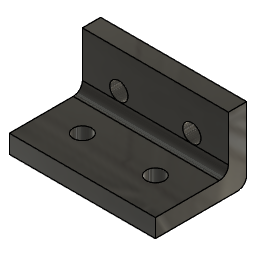
Fully Assembled English Wheel (Autodesk Fusion 360 archive; units mm, degrees)
design "Clamp/Mount Bracket"
Autodesk Fusion 360 part; units mm, degrees
sketch "Sketch1" plane through (0, 0, 0) normal (0, 1, 0) x (1, 0, 0)
  line L0 (50.8, 25.4) -> (-50.8, 25.4)
  line L1 (-50.8, 25.4) -> (-50.8, -25.4)
  line L2 (-50.8, -25.4) -> (50.8, -25.4)
  line L3 (50.8, -25.4) -> (50.8, 25.4)
  line L4 (0, 0) -> (25.4, 0) construction
  line L5 (0, 0) -> (-25.4, 0) construction
  circle A0 centre (-25.4, 0) radius 6.35
  circle A1 centre (25.4, 0) radius 6.35
  dimension "d3" = 101.6
  dimension "d4" = 50.8
  dimension "d5" = 25.4
  dimension "d7" = 12.7
  dimension "d8" = 12.7
  constraint horizontal L0
  constraint perpendicular L0 L1
  constraint parallel L0 L2
  constraint parallel L1 L3
  constraint coincident L4.start L5.start
  constraint horizontal L4
  constraint parallel L4 L5
  constraint coincident L5.end A0.centre
  constraint coincident L4.end A1.centre
  measures "d3" distance of L1.end L2.end
  measures "d4" distance of L0.end L1.end
  measures "d5" distance of L4.start L4.end
  measures "d7" diameter of A0
  measures "d8" diameter of A1
extrude "Extrude1" add sketch "Sketch1" along normal blind 12.7 makes body 1
sketch "Sketch2" plane through (0, 0, 0) normal (0, -1, 0) x (1, 0, 0)
  circle A0 centre (-25.4, 0) radius 6.35
  circle A1 centre (25.4, 0) radius 6.35
  line L0 (50.8, -25.4) -> (50.8, 25.4)
  line L1 (50.8, 25.4) -> (-50.8, 25.4)
  line L2 (-50.8, 25.4) -> (-50.8, -25.4)
  line L3 (-50.8, -25.4) -> (50.8, -25.4)
  line L4 (-50.8, -25.4) -> (50.8, -25.4)
  line L5 (50.8, -25.4) -> (50.8, -12.7)
  line L6 (50.8, -12.7) -> (-50.8, -12.7)
  line L7 (-50.8, -12.7) -> (-50.8, -25.4)
  dimension "d11" = 101.6
  dimension "d12" = 12.7
  constraint horizontal L4
  constraint vertical L5
  constraint horizontal L6
  constraint vertical L7
  constraint coincident L2.end L3.start
  measures "d11" distance of L2.end L0.start
  measures "d12" distance of L0.start L5.end
extrude "Extrude2" add sketch "Sketch2" along normal blind 50.8 contours L0 L2 L3 L4 L5 L6 L7 bodies 1
sketch "Sketch3" plane through (0, 0, -12.7) normal (0, 0, 1) x (-1, 0, 0)
  line L0 (-50.8, 0) -> (50.8, 0)
  line L1 (50.8, 0) -> (50.8, 50.8)
  line L2 (50.8, 50.8) -> (-50.8, 50.8)
  line L3 (-50.8, 50.8) -> (-50.8, 0)
  line L4 (0, 0) -> (0, 50.8) construction
  line L5 (0, 25.4) -> (-25.4, 25.4) construction
  line L6 (0, 25.4) -> (25.4, 25.4) construction
  circle A0 centre (25.4, 25.4) radius 6.35
  circle A1 centre (-25.4, 25.4) radius 6.35
  dimension "d15" = 25.4
  dimension "d16" = 25.4
  dimension "d17" = 12.7
  dimension "d18" = 12.7
  constraint coincident L4.start origin
  constraint midpoint L2 L4.end
  constraint midpoint L4 L5.start
  constraint perpendicular L4 L5
  constraint perpendicular L4 L6
  constraint coincident L6.end A0.centre
  constraint coincident L5.end A1.centre
  measures "d15" distance of L5.start L5.end
  measures "d16" distance of L5.start L6.end
  measures "d17" diameter of A0
  measures "d18" diameter of A1
extrude "Extrude3" cut sketch "Sketch3" against normal blind 43.18 contours A0 | A1 bodies 1
fillet "Fillet1" radius 6.35 2 edges at (0, 0, -12.7) (0, 12.7, -25.4) on bodies 1
copy_body "Body->Comp1" bodies 1 removing the originals makes body 2 in component "Clamp/Mount Bracket"
component "Clamp/Mount Bracket" placed x (1, 0, 0) y (0, 1, 0) z (0, 0, 1) at (0, 0, 0)
equation "d7 = ( 1 / 2 ) * 1 in"
equation "d8 = ( 1 / 2 ) * 1 in"
equation "d9 = ( 1 / 2 ) * 1 in"
equation "d17 = ( 1 / 2 ) * 1 in"
equation "d18 = ( 1 / 2 ) * 1 in"
equation "d22 = ( 1 / 4 ) * 1 in"

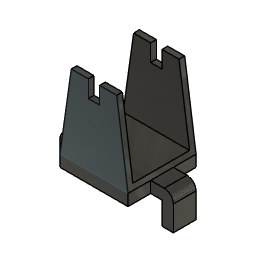
design "Lower Anvil Holder"
Autodesk Fusion 360 part; units mm, degrees
sketch "Sketch1" plane through (0, 0, 0) normal (0, 1, 0) x (1, 0, 0)
  line L0 (19.05, 22.225) -> (-19.05, 22.225)
  line L1 (-19.05, 22.225) -> (-19.05, -22.225)
  line L2 (-19.05, -22.225) -> (19.05, -22.225)
  line L3 (19.05, -22.225) -> (19.05, 22.225)
  line L4 (0, -22.225) -> (12.7, -22.225)
  line L5 (0, -22.225) -> (-12.7, -22.225)
  line L6 (-19.05, 22.225) -> (-12.7, -22.225)
  line L7 (12.7, -22.225) -> (19.05, 22.225)
  line L8 (0, -22.225) -> (3.175, -22.225)
  line L9 (0, -22.225) -> (-3.175, -22.225)
  line L10 (-3.175, -22.225) -> (-3.175, -12.7)
  line L11 (3.175, -22.225) -> (3.175, -12.7)
  line L12 (-3.175, -12.7) -> (3.175, -12.7)
  dimension "d1" = 38.1
  dimension "d2" = 44.45
  constraint horizontal L0
  constraint perpendicular L0 L1
  constraint parallel L0 L2
  constraint parallel L1 L3
  constraint midpoint L2 L4.start
  constraint parallel L2 L4
  constraint coincident L2 L5.end
  constraint coincident L4 L8.end
  constraint coincident L5 L9.end
  constraint perpendicular L5 L10
  constraint perpendicular L2 L11
  measures "d1" distance of L1.end L2.end
  measures "d2" distance of L0.end L1.end
extrude "Extrude1" add sketch "Sketch1" along normal blind 38.1 contours L0 L2 L4 L5 L6 L7 L10 L11 L12 makes body 1
sketch "Sketch2" plane through (0, 0, 0) normal (0, -1, 0) x (1, 0, 0)
  line L0 (-3.175, 12.7) -> (-3.175, 22.225)
  line L1 (-3.175, 22.225) -> (-12.7, 22.225)
  line L2 (-12.7, 22.225) -> (-19.05, -22.225)
  line L3 (-19.05, -22.225) -> (19.05, -22.225)
  line L4 (19.05, -22.225) -> (12.7, 22.225)
  line L5 (12.7, 22.225) -> (3.175, 22.225)
  line L6 (3.175, 22.225) -> (3.175, 12.7)
  line L7 (3.175, 12.7) -> (-3.175, 12.7)
sketch "Sketch3" plane through (0, 0, 0) normal (1, 0, 0) x (0, 1, 0)
  line L0 (0, 0) -> (38.1, 0) construction
  line L1 (19.05, 0) -> (19.05, -22.225) construction
  line L2 (19.05, 0) -> (19.05, 22.225) construction
  line L3 (19.05, 22.225) -> (3.175, 22.225) construction
  line L4 (3.175, 22.225) -> (34.925, 22.225)
  line L5 (34.925, 22.225) -> (34.925, -19.05)
  line L6 (34.925, -19.05) -> (3.175, -19.05)
  line L7 (3.175, -19.05) -> (3.175, 22.225)
  dimension "d13" = 31.75
  dimension "d14" = 41.275
  constraint coincident L0.start origin
  constraint horizontal L0
  constraint midpoint L0 L1.start
  constraint perpendicular L0 L1
  constraint perpendicular L0 L2
  constraint perpendicular L2 L3
  constraint horizontal L4
  constraint vertical L5
  constraint horizontal L6
  constraint vertical L7
  measures "d13" distance of L3.end L4.end
  measures "d14" distance of L3.end L6.end
extrude "Extrude2" cut sketch "Sketch3" along normal blind 76.2 and the other way blind 60.96 bodies 1
extrude "Extrude3" add 1 faces at (6.35, 12.7, -22.225) along direction (0, 0, -1) blind 6.35 on bodies 1 bodies 1
sketch "Sketch4" plane through (19.05, 0, 0) normal (1, 0, 0) x (0, 1, 0)
  line L0 (38.1, -22.225) -> (0, -22.225)
  line L1 (0, -22.225) -> (0, -28.575)
  line L2 (0, -28.575) -> (38.1, -28.575)
  line L3 (38.1, -28.575) -> (38.1, -22.225)
  line L4 (19.05, -22.225) -> (25.4, -22.225)
  line L5 (19.05, -22.225) -> (12.7, -22.225)
  line L6 (12.7, -22.225) -> (12.7, -28.575)
  line L7 (25.4, -22.225) -> (25.4, -28.575)
  line L8 (12.7, -28.575) -> (25.4, -28.575)
  dimension "d21" = 6.35
  constraint midpoint L0 L4.start
  constraint parallel L0 L4
  constraint parallel L0 L5
  constraint coincident L2 L6.end
  constraint perpendicular L2 L6
  constraint coincident L2 L7.end
  constraint perpendicular L2 L7
  measures "d21" distance of L4.start L4.end
extrude "Extrude4" add sketch "Sketch4" along normal blind 12.7 contours L0 L2 L4 L5 L6 L7 L8 bodies 1
extrude "Extrude5" add 1 faces at (31.75, 21.1667, -26.4583) along direction (-1, 0, 0) blind 63.5 on bodies 1 bodies 1
copy_body "Body->Comp1" bodies 1 removing the originals makes body 2 in component "Lower Anvil Holder"
sketch "Sketch5" plane through (0, 0, -28.575) normal (0, 0, -1) x (1, 0, 0)
  line L0 (19.05, -12.7) -> (19.05, 0)
  line L1 (19.05, 0) -> (-19.05, 0)
  line L2 (-19.05, 0) -> (-19.05, -12.7)
  line L3 (-19.05, -12.7) -> (-31.75, -12.7)
  line L4 (-31.75, -12.7) -> (-31.75, -25.4)
  line L5 (-31.75, -25.4) -> (-19.05, -25.4)
  line L6 (-19.05, -25.4) -> (-19.05, -38.1)
  line L7 (-19.05, -38.1) -> (19.05, -38.1)
  line L8 (19.05, -38.1) -> (19.05, -25.4)
  line L9 (19.05, -25.4) -> (31.75, -25.4)
  line L10 (31.75, -25.4) -> (31.75, -12.7)
  line L11 (31.75, -12.7) -> (19.05, -12.7)
  line L12 (31.75, -19.05) -> (25.4, -19.05) construction
  line L13 (25.4, -19.05) -> (25.4, -12.7)
  line L14 (25.4, -19.05) -> (25.4, -25.4)
  line L15 (-31.75, -19.05) -> (-25.4, -19.05) construction
  line L16 (-25.4, -19.05) -> (-25.4, -12.7)
  line L17 (-25.4, -19.05) -> (-25.4, -25.4)
  dimension "d27" = 6.35
  dimension "d28" = 6.35
  constraint midpoint L10 L12.start
  constraint perpendicular L10 L12
  constraint midpoint L11 L13.end
  constraint midpoint L9 L14.end
  constraint midpoint L4 L15.start
  constraint perpendicular L4 L15
  constraint midpoint L3 L16.end
  constraint midpoint L5 L17.end
  measures "d27" distance of L12.start L12.end
  measures "d28" distance of L15.start L15.end
extrude "Extrude1'" add sketch "Sketch5" along normal blind 12.7 contours L9 L10 L11 L13 L14 | L3 L4 L5 L16 L17 bodies 2 in component "Lower Anvil Holder"
fillet "Fillet1" radius 5.08 2 edges at (-31.75, 19.05, -22.225) (31.75, 19.05, -22.225) on bodies 2 in component "Lower Anvil Holder"
component "Lower Anvil Holder" placed x (1, 0, 0) y (0, 1, 0) z (0, 0, 1) at (0, 0, 0)

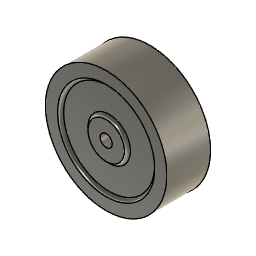
design "Upper Rolling Wheel"
Autodesk Fusion 360 part; units mm, degrees
sketch "Sketch1" plane through (0, 0, 0) normal (0, 1, 0) x (1, 0, 0)
  circle A0 centre (0, 0) radius 63.5
  circle A1 centre (0, 0) radius 6.35
  constraint coincident A0.centre A1.centre
  constraint concentric A0 A1
extrude "Extrude1" add sketch "Sketch1" along normal blind 45.72 makes body 1
sketch "Sketch2" plane through (0, 0, 0) normal (0, -1, 0) x (1, 0, 0)
  circle A0 centre (0, 0) radius 6.35
  circle A1 centre (0, 0) radius 63.5
  circle A2 centre (0, 0) radius 50.8
  circle A3 centre (0, 0) radius 19.05
  dimension "d5" = 101.6
  dimension "d6" = 38.1
  constraint concentric A0 A2
  constraint concentric A2 A3
  measures "d5" diameter of A2
  measures "d6" diameter of A3
extrude "Extrude2" cut sketch "Sketch2" against normal blind 3.175 contours A2 bodies 1
sketch "Sketch3" plane through (0, 45.72, 0) normal (0, 1, 0) x (-1, 0, 0)
  circle A0 centre (0, 0) radius 6.35
  circle A1 centre (0, 0) radius 63.5
  circle A2 centre (0, 0) radius 50.8
  circle A3 centre (0, 0) radius 19.05
  dimension "d9" = 101.6
  dimension "d10" = 38.1
  constraint concentric A0 A2
  constraint concentric A2 A3
  measures "d9" diameter of A2
  measures "d10" diameter of A3
extrude "Extrude3" cut sketch "Sketch3" against normal blind 3.175 contours A2 bodies 1
fillet "Fillet1" radius 3.175 2 edges at (17.7608, 42.545, -6.8888) (47.3622, 42.545, 18.3701) on bodies 1
fillet "Fillet2" radius 3.175 2 edges at (-17.7608, 3.175, -6.8888) (-47.3622, 3.175, 18.3701) on bodies 1
copy_body "Body->Comp1" bodies 1 removing the originals makes body 2 in component "Rolling Wheel"
component "Rolling Wheel" placed x (1, 0, 0) y (0, 1, 0) z (0, 0, 1) at (0, 0, 0)
equation "d7 = ( -1 / 4 / 2 ) * 1 in"
named bodies: "Rolling Wheel"
